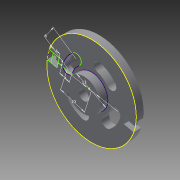
# Autodesk Inventor part: MotorFenek
Saved by Autodesk Inventor 2015 (Build 190159000, 159)
## iProperties
Created: 2014-08-26
Part Number: MotorFenek
Material: Generic
Document SubType Name: Modeling
Designer: laca
Density: 1 g/cm^3
Appearance: Default
Mass: 2.78751 g
Surface Area: 25.132 cm^2
Volume: 2.78751 cm^3
Author: laca
Autodesk Inventor part; units mm, degrees
ref_plane "YZ Plane" through (0, 0, 0) normal (1, 0, 0) x (0, 1, 0)
ref_plane "XZ Plane" through (0, 0, 0) normal (0, 1, 0) x (-1, 0, 0)
ref_plane "XY Plane" through (0, 0, 0) normal (0, 0, 1) x (1, 0, 0)
sketch "Sketch2" plane through (0, 0, 0) normal (0, 0, 1) x (1, 0, 0)
  circle A0 centre (0, 0) radius 17.8
  dimension "d0" = 35.6
  constraints: 1 centre point, 1 coincident
  measures "d0" diameter of A0
extrude "Extrusion1" add sketch "Sketch2" along normal blind 3
sketch "Sketch3" plane through (0, 0, 3) normal (0, 0, 1) x (1, 0, 0)
  circle A0 centre (0, 0) radius 6.5
  circle A1 centre (0, 0) radius 2
  arc A2 (-6.1065, 7.919) -> (-9.5399, 2.9985) centre (0, 0) ccw construction
  arc A3 (-7.3277, 9.5029) -> (-11.4478, 3.5982) centre (0, 0) ccw
  arc A4 (-4.8852, 6.3352) -> (-7.6319, 2.3988) centre (0, 0) ccw
  arc A5 (-4.8852, 6.3352) -> (-7.3277, 9.5029) centre (-6.1065, 7.919) ccw
  arc A6 (-11.4478, 3.5982) -> (-7.6319, 2.3988) centre (-9.5399, 2.9985) ccw
  circle A7 centre (0, 0) radius 17.8 projected
  line L0 (0, 0) -> (-13.3383, 3.0709)
  line L1 (-16.7877, 5.9173) -> (-12.8896, 5.0199)
  line L2 (-12.8896, 5.0199) -> (-13.3383, 3.0709)
  line L3 (-17.6851, 2.0193) -> (-13.7871, 1.1219)
  line L4 (-13.7871, 1.1219) -> (-13.3383, 3.0709)
  arc A8 (-16.7877, 5.9173) -> (-17.6851, 2.0193) centre (0, 0) ccw
  arc A9 (-15.2021, 5.563) -> (-16.1032, 1.6551) centre (0, 0) ccw
  line L5 (-16.7877, 5.9173) -> (-15.2057, 5.5531)
  line L6 (-16.1032, 1.6551) -> (-17.6851, 2.0193)
  dimension "d3" = 13
  dimension "d4" = 4
  dimension "d18" = 10
  dimension "d20" = 4
  dimension "d26" = 4
  dimension "d27" = 2
  dimension "d33" = 6
  constraints: 15 point on circle, 14 end point, 9 centre point, 5 coincident, 4 tangent, 2 parallel, 2 point on line, 2 symmetric about line, 1 perpendicular, 2 other
  measures "d3" diameter of A0
  measures "d4" diameter of A1
  measures "d18" distance of point (0, 0) A2.end
  measures "d20" distance of A4.end A3.end
  measures "d26" distance of L1.start L1.end
  measures "d27" distance of L0.end L1.end
  measures "d33" distance of A2.end A2.start
extrude "Extrusion2" add sketch "Sketch3" along normal blind 3 contours A0
extrude "Extrusion3" cut sketch "Sketch3" against normal through all contours A1
extrude "Extrusion5" cut sketch "Sketch3" against normal blind 3 contours A6 L0 | L0 A6 A3 A5 A4
pattern_circular "Circular Pattern1" count 4 over 360 about axis through (0, 0, 3) along (0, 0, 1) of "Extrusion5"
extrude "Extrusion6" cut sketch "Sketch3" against normal blind 2 contours L4 L3 A9 L1 L2 | A9 L3 A7 L1
extrude "Extrusion7" cut sketch "Sketch3" against normal through all contours A9 L3 A7 L1
pattern_circular "Circular Pattern3" count 2 over 360 about axis through (0, 0, 3) along (0, 0, 1) of "Extrusion6", "Extrusion7"
body "Solid1"
